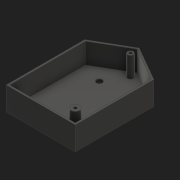
# Autodesk Inventor part: AC03
Saved by Autodesk Inventor 2017 (Build 210142000, 142)
## iProperties
Created: 2019-08-28
Part Number: AC03
Material: ABS Plastic
Document SubType Name: Modeling
Designer: Dell
Density: 1.06 g/cm^3
Appearance: Smooth - Black
Author: Dell
Autodesk Inventor part; units mm, degrees
ref_plane "YZ Plane" through (0, 0, 0) normal (1, 0, 0) x (0, 1, 0)
ref_plane "XZ Plane" through (0, 0, 0) normal (0, 1, 0) x (-1, 0, 0)
ref_plane "XY Plane" through (0, 0, 0) normal (0, 0, 1) x (1, 0, 0)
sketch "Sketch1" plane through (0, 0, 0) normal (0, 0, 1) x (1, 0, 0)
  line L0 (0, 68.1273) -> (59, 34.0637)
  line L1 (59, 34.0637) -> (59, -34.0637)
  line L2 (59, -34.0637) -> (0, -68.1273)
  line L3 (0, -68.1273) -> (-59, -34.0637)
  line L4 (-59, -34.0637) -> (-59, 34.0637)
  line L5 (-59, 34.0637) -> (0, 68.1273)
  line L6 (-59, -34.0637) -> (-59, -100)
  line L7 (-59, -100) -> (59, -100)
  line L8 (59, -100) -> (59, -34.0637)
  point P0 (0, 0)
  point P1 (0, 0)
  dimension "d0" = 118
  dimension "d1" = 100
  constraints: 18 end point, 2 perpendicular, 1 coincident, 1 vertical, 1 vertical alignment, 13 other
  measures "d0" distance between parallel lines of L1 L4
  measures "d1" distance from line of L7 point (0, 0)
extrude "Extrusion1" add sketch "Sketch1" along normal blind 5
sketch "Sketch2" plane through (0, 0, 5) normal (0, 0, 1) x (1, 0, 0)
  line L0 (59, -100) -> (59, 34.0637) projected
  line L1 (59, 34.0637) -> (0, 68.1273) projected
  line L2 (0, 68.1273) -> (-59, 34.0637) projected
  line L3 (-59, 34.0637) -> (-59, -100) projected
  line L4 (-59, -100) -> (59, -100) projected
  line L5 (-56, 32.3316) -> (0, 64.6632)
  line L6 (0, 64.6632) -> (56, 32.3316)
  line L7 (56, 32.3316) -> (56, -97)
  line L8 (56, -97) -> (-56, -97)
  line L9 (-56, -97) -> (-56, 32.3316)
  point P0 (0, 0)
  dimension "d4" = 3
  constraints: 10 end point, 4 other
  measures "d4" distance between parallel lines of L2 L5
extrude "Extrusion2" add sketch "Sketch2" along normal blind 35
sketch "Sketch3" plane through (0, 0, 0) normal (0, 0, -1) x (-1, 0, 0)
  circle A0 centre (0, 53.1273) radius 2.5
  circle A1 centre (-34, -75) radius 2.5
  line L0 (59, -100) -> (-59, -100) projected
  line L1 (-59, -100) -> (-59, 34.0637) projected
  point P0 (0, 0)
  point P1 (0, 68.1273)
  dimension "d7" = 5
  dimension "d8" = 5
  dimension "d9" = 25
  dimension "d10" = 25
  dimension "d11" = 15
  constraints: 2 centre point, 1 vertical alignment
  measures "d7" diameter of A0
  measures "d8" diameter of A1
  measures "d9" distance from line of L0 A1.centre
  measures "d10" distance from line of A1.centre L1
  measures "d11" distance of A0.centre point (0, 68.127)
extrude "Extrusion3" cut sketch "Sketch3" against normal through all
sketch "Sketch4" plane through (0, 0, 0) normal (0, 0, -1) x (-1, 0, 0)
  circle A0 centre (19.799, 19.799) radius 5
  line L0 (59, 34.0637) -> (59, -100) projected
  line L1 (59, -100) -> (-59, -100) projected
  point P0 (0, 0)
  dimension "d14" = 10
  dimension "d15" = 39.201
  dimension "d16" = 119.799
  constraints: 1 centre point
  measures "d14" diameter of A0
  measures "d15" distance from line of L0 A0.centre
  measures "d16" distance from line of L1 A0.centre
extrude "Extrusion4" cut sketch "Sketch4" against normal through all
sketch "Sketch5" plane through (0, 0, 5) normal (0, 0, 1) x (1, 0, 0)
  circle A0 centre (0, 53.1273) radius 2.5 projected
  circle A1 centre (0, 53.1273) radius 5
  circle A2 centre (34, -75) radius 2.5 projected
  circle A3 centre (34, -75) radius 7.5
  point P0 (0, 0)
  dimension "d19" = 10
  dimension "d20" = 15
  constraints: 2 centre point, 2 coincident
  measures "d19" diameter of A1
  measures "d20" diameter of A3
extrude "Extrusion5" add sketch "Sketch5" along normal up to surface (35 mm away) from surface at 0
body "Solid1"
